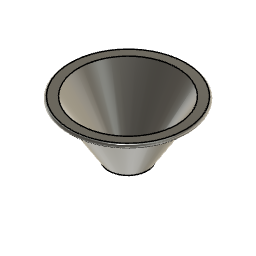
bowl (Autodesk Fusion 360 design; units mm, degrees)
Autodesk Fusion 360 part; units mm, degrees
sketch "Sketch1" plane through (0, 0, 0) normal (0, 1, 0) x (1, 0, 0) in component "bowl"
  line L0 (0, 0) -> (15, 0)
  line L1 (15, 0) -> (40, -40)
  line L2 (40, -40) -> (45, -40)
  line L3 (0, -3) -> (13.3373, -3)
  line L4 (13.3373, -3) -> (38.3373, -43)
  line L5 (38.3373, -43) -> (45, -43)
  arc A0 (45, -43) -> (45, -40) centre (45, -41.5) ccw
  line L6 (0, -3) -> (0, 0)
  dimension "d1" = 3
  constraint coincident L0.start L6.end
  constraint horizontal L0
  constraint parallel L0 L2
  constraint tangent L2 A0
  constraint perpendicular L0 L6
revolve "Revolve1" add sketch "Sketch1" angle 360 about axis through (0, 0, 1.75) along (0, 0, 1) in component "bowl"
component "bowl" placed x (1, 0, 0) y (0, 1, 0) z (0, 0, 1) at (0, 0, 0)
